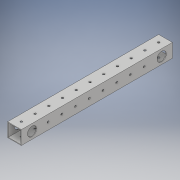
# Autodesk Inventor part: Support Pivs 11
Saved by Autodesk Inventor 2018 (Build 220112000, 112)
## iProperties
Created: 2018-01-22
Part Number: Support Pivs 11
Material: Generic
Document SubType Name: Modeling
Designer: lopez.xavier
Density: 1 g/cm^3
Appearance: Default
Author: lopez.xavier
Autodesk Inventor part; units mm, degrees
ref_plane "YZ Plane" through (0, 0, 0) normal (1, 0, 0) x (0, 1, 0)
ref_plane "XZ Plane" through (0, 0, 0) normal (0, 1, 0) x (-1, 0, 0)
ref_plane "XY Plane" through (0, 0, 0) normal (0, 0, 1) x (1, 0, 0)
sketch "Sketch1" plane through (0, 0, 0) normal (0, 0, 1) x (1, 0, 0)
  line L0 (0, 0) -> (25.4, 0)
  line L1 (25.4, 0) -> (25.4, 25.4)
  line L2 (25.4, 25.4) -> (0, 25.4)
  line L3 (0, 25.4) -> (0, 0)
  dimension "d0" = 25.4
  dimension "d1" = 25.4
  constraints: 8 end point, 2 parallel, 1 horizontal, 1 perpendicular
  measures "d0" distance of L2.end L1.end
  measures "d1" distance of L1.end L0.end
extrude "Extrusion1" add sketch "Sketch1" along normal blind 279.4
shell "Shell1" thickness 1.143 removed faces 2 at (8.4667, 16.9333, 0) at (8.4667, 16.9333, 279.4)
sketch "Sketch2" plane through (25.4, 0, 0) normal (1, 0, 0) x (0, 0, -1)
  circle A0 centre (-259.5499, 12.7) radius 8.5725
  line L0 (-279.4, 0) -> (-279.4, 25.4) projected
  line L1 (0, 25.4) -> (-279.4, 25.4) projected
  circle A1 centre (-19.8501, 12.7) radius 8.5725
  line L2 (0, 0) -> (0, 25.4) projected
  dimension "d5" = 17.145
  dimension "d6" = 19.8501
  dimension "d7" = 12.7
  dimension "d8" = 17.145
  dimension "d9" = 19.8501
  dimension "d10" = 12.7
  constraints: 2 centre point
  measures "d5" diameter of A0
  measures "d6" distance from line of L0 A0.centre
  measures "d7" distance from line of L1 A0.centre
  measures "d8" diameter of A1
  measures "d9" distance from line of L2 A1.centre
  measures "d10" distance from line of L1 A1.centre
extrude "Extrusion2" cut sketch "Sketch2" against normal blind 279.4
sketch "Sketch3" plane through (0, 25.4, 0) normal (0, 1, 0) x (1, 0, 0)
  circle A0 centre (12.7, -12.7) radius 1.905
  line L0 (25.4, 0) -> (0, 0) projected
  line L1 (0, 0) -> (0, -279.4) projected
  circle A1 centre (12.7, -38.1) radius 1.905
  circle A2 centre (12.7, -63.5) radius 1.905
  circle A3 centre (12.7, -88.9) radius 1.905
  circle A4 centre (12.7, -114.3) radius 1.905
  circle A5 centre (12.7, -139.7) radius 1.905
  circle A6 centre (12.7, -165.1) radius 1.905
  circle A7 centre (12.7, -190.5) radius 1.905
  circle A8 centre (12.7, -215.9) radius 1.905
  circle A9 centre (12.7, -241.3) radius 1.905
  circle A10 centre (12.7, -266.7) radius 1.905
  dimension "d13" = 3.81
  dimension "d14" = 12.7
  dimension "d15" = 12.7
  dimension "d18" = 25.4
  constraints: 11 centre point, 1 vertical, 20 other
  measures "d13" diameter of A0
  measures "d14" distance from line of L0 A0.centre
  measures "d15" distance from line of L1 A0.centre
  measures "d18" distance of A0.centre A1.centre
extrude "Extrusion3" cut sketch "Sketch3" against normal blind 279.4
sketch "Sketch4" plane through (25.4, 0, 0) normal (1, 0, 0) x (0, 0, -1)
  circle A0 centre (-255.4224, 12.7) radius 1.905
  line L0 (0, 25.4) -> (-279.4, 25.4) projected
  circle A1 centre (-259.5499, 12.7) radius 8.5725 projected
  circle A2 centre (-230.0224, 12.7) radius 1.905
  circle A3 centre (-204.6224, 12.7) radius 1.905
  circle A4 centre (-179.2224, 12.7) radius 1.905
  circle A5 centre (-153.8224, 12.7) radius 1.905
  circle A6 centre (-128.4224, 12.7) radius 1.905
  circle A7 centre (-103.0224, 12.7) radius 1.905
  circle A8 centre (-77.6224, 12.7) radius 1.905
  circle A9 centre (-52.2224, 12.7) radius 1.905
  point P0 (0, 0)
  dimension "d25" = 3.81
  dimension "d26" = 12.7
  dimension "d27" = 4.1275
  dimension "d30" = 25.4
  constraints: 9 centre point, 1 horizontal, 16 other
  measures "d25" diameter of A0
  measures "d26" distance from line of L0 A0.centre
  measures "d27" distance of A1.centre A0.centre
  measures "d30" distance of A0.centre A2.centre
extrude "Extrusion4" cut sketch "Sketch4" against normal blind 279.4 contours A2 | A3 | A4 | A5 | A6 | A7 | A8 | A9
equation "\"d8\" = d5"
equation "\"d9\" = d6"
equation "\"d10\" = d7"
body "Solid1"
